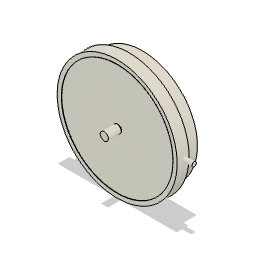
movements (Autodesk Fusion 360 design; units mm, degrees)
Autodesk Fusion 360 part; units mm, degrees
sketch "Sketch1" plane through (0, 0, 0) normal (0, 0, 1) x (1, 0, 0) in component "nh38"
  circle A0 centre (0, 0) radius 14.73
  dimension "d1" = 29.46
  constraint coincident A0.centre origin
  measures "d1" diameter of A0
extrude "Extrude1" add sketch "Sketch1" against normal blind 2.94 makes body 1 in component "nh38"
sketch "Sketch2" plane through (0, 0, -2.94) normal (0, 0, -1) x (-1, 0, 0) in component "nh38"
  circle A0 centre (0, 0) radius 14.73
  circle A1 centre (0, 0) radius 13.5
  dimension "d4" = 27
  constraint concentric A0 A1
  measures "d4" diameter of A1
extrude "Extrude2" add sketch "Sketch2" along normal blind 3.28 contours A1 bodies 1 in component "nh38"
sketch "Sketch3" plane through (0, 0, 0) normal (0, 0, 1) x (1, 0, 0) in component "nh38"
  circle A0 centre (0, 0) radius 14.73
  circle A1 centre (0, 0) radius 0.75
  dimension "d7" = 1.5
  constraint concentric A0 A1
  measures "d7" diameter of A1
extrude "Extrude3" add sketch "Sketch3" along normal blind 1.18 contours A1 bodies 1 in component "nh38"
sketch "Sketch4" plane through (0, 0, 0) normal (0, 0, 1) x (1, 0, 0) in component "nh38"
  circle A0 centre (0, 0) radius 0.75
  circle A1 centre (0, 0) radius 14.73
  circle A2 centre (0, 0) radius 0.445
  dimension "d10" = 0.89
  constraint concentric A0 A2
  measures "d10" diameter of A2
extrude "Extrude4" add sketch "Sketch4" along normal blind 1.77 contours A2 bodies 1 in component "nh38"
sketch "Sketch5" plane through (0, 0, 0) normal (0, 0, 1) x (1, 0, 0) in component "nh38"
  circle A0 centre (0, 0) radius 0.75
  circle A1 centre (0, 0) radius 14.73
  circle A2 centre (0, 0) radius 0.1075
  dimension "d13" = 0.215
  constraint concentric A0 A2
  measures "d13" diameter of A2
extrude "Extrude5" add sketch "Sketch5" along normal blind 2.31 contours A2 bodies 1 in component "nh38"
sketch "Sketch6" plane through (0, 0, 0) normal (0, 0, 1) x (1, 0, 0) in component "nh38"
  circle A0 centre (0, 0) radius 0.75
  circle A1 centre (0, 0) radius 14.73
  circle A2 centre (0, 0) radius 1
  dimension "d16" = 2
  constraint coincident A0.centre A1.centre
  measures "d16" diameter of A2
extrude "Extrude6" add sketch "Sketch6" along normal blind 3.16 separate body contours A0 | A2 makes body 2 in component "nh38"
sketch "Sketch1 (2)" plane through (0, 0, 0) normal (0, 0, 1) x (1, 0, 0)
  circle A0 centre (0, 0) radius 0.75
  circle A1 centre (0, 0) radius 14.73
  circle A2 centre (0, 0) radius 13.7
  circle A3 centre (0, 0) radius 1
  dimension "d19" = 27.4
  dimension "d20" = 2
  constraint concentric A0 A2
  constraint concentric A2 A3
  measures "d19" diameter of A2
  measures "d20" diameter of A3
extrude "Extrude7" cut sketch "Sketch1 (2)" against normal blind 0.1 contours A2 bodies 1 in component "nh38"
sketch "Sketch2 (2)" plane through (0, 0, 0) normal (1, 0, 0) x (0, 0, -1) in component "nh38"
  line L0 (0, 0) -> (1.92, 0) construction
  circle A0 centre (1.92, 0) radius 0.55
  dimension "d23" = 1.92
  dimension "d24" = 1.1
  constraint coincident L0.start origin
  constraint horizontal L0
  constraint coincident L0.end A0.centre
  measures "d23" distance of L0.start L0.end
  measures "d24" diameter of A0
extrude "Extrude8" add sketch "Sketch2 (2)" along normal blind 17 separate body makes body 3 in component "nh38"
component "seiko-tmi" placed x (1, 0, 0) y (0, 1, 0) z (0, 0, 1) at (0, 0, 0)
component "nh38" placed x (1, 0, 0) y (0, 1, 0) z (0, 0, 1) at (0, 0, 0) in component "seiko-tmi"
equation "d5 = 5.32 mm - 2.94 mm + 0.4 mm + 0.5 mm"
equation "d8 = 0.4 mm + 0.78 mm"
equation "d11 = 0.4 mm + 1.37 mm"
equation "d14 = 0.4 mm + 1.91 mm"
equation "d17 = 0.4 mm + 2.31 mm + 0.45 mm"
named bodies: "movement", "movement-to-glass-distance", "stemm"
